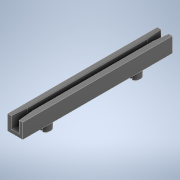
# Autodesk Inventor part: RDC-250
Saved by Autodesk Inventor 2021 (Build 250183000, 183)
## iProperties
Created: 2021-01-15
Part Number: RDC-250
Material: Nylon 6/6
Document SubType Name: Modeling
Designer: dimercur
Density: 1.13 g/cm^3
Appearance: Lisse - Noir
Author: dimercur
Autodesk Inventor part; units mm, degrees
ref_plane "YZ Plane" through (0, 0, 0) normal (1, 0, 0) x (0, 1, 0)
ref_plane "XZ Plane" through (0, 0, 0) normal (0, 1, 0) x (-1, 0, 0)
ref_plane "XY Plane" through (0, 0, 0) normal (0, 0, 1) x (1, 0, 0)
sketch "Esquisse1" plane through (0, 0, 0) normal (0, 1, 0) x (-1, 0, 0)
  line L0 (3.2, 31.75) -> (-3.2, 31.75)
  line L1 (-3.2, 31.75) -> (-3.2, -31.75)
  line L2 (-3.2, -31.75) -> (3.2, -31.75)
  line L3 (3.2, -31.75) -> (3.2, 31.75)
  point P0 (0, 0)
  dimension "d0" = 63.5
  dimension "d1" = 6.4
  dimension "d2" = 3.2
  dimension "d3" = 31.75
  constraints: 8 end point, 2 parallel, 1 horizontal, 1 perpendicular
  measures "d0" distance of L2.end L0.start
  measures "d1" distance of L0.start L0.end
  measures "d2" horizontal distance of point (0, 0) L0.start
  measures "d3" vertical distance of L0.start point (0, 0)
extrude "Extrusion1" add sketch "Esquisse1" along normal blind 6.4
sketch "Esquisse2" plane through (0, 6.4, 0) normal (0, 1, 0) x (1, 0, 0)
  line L0 (-3.2, -31.75) -> (3.2, -31.75) projected
  line L1 (-1.65, -31.75) -> (-1, -25.35)
  line L2 (-1, -25.35) -> (-1, 25.35)
  line L3 (-1, 25.35) -> (-1.65, 31.75)
  line L4 (3.2, 31.75) -> (-3.2, 31.75) projected
  line L5 (-1.65, 31.75) -> (1.65, 31.75)
  line L6 (1.65, 31.75) -> (1, 25.35)
  line L7 (1, 25.35) -> (1, -25.35)
  line L8 (1, -25.35) -> (1.65, -31.75)
  line L9 (1.65, -31.75) -> (-1.65, -31.75)
  point P0 (0, 0)
  dimension "d6" = 3.3
  dimension "d7" = 3.3
  dimension "d8" = 1.65
  dimension "d9" = 1.65
  dimension "d10" = 2
  dimension "d11" = 1
  dimension "d12" = 6.4
  dimension "d13" = 6.4
  dimension "d14" = 6.4
  dimension "d15" = 6.4
  constraints: 16 end point, 2 perpendicular, 2 point on line, 1 horizontal, 1 parallel
  measures "d6" distance of L8.end L1.start
  measures "d7" distance of L5.end L3.end
  measures "d8" horizontal distance of point (0, 0) L3.end
  measures "d9" horizontal distance of point (0, 0) L1.start
  measures "d10" distance between parallel lines of L7 L2
  measures "d11" horizontal distance of point (0, 0) L1.end
  measures "d12" vertical distance of L1.start L1.end
  measures "d13" vertical distance of L8.end L7.end
  measures "d14" vertical distance of L3.end L2.end
  measures "d15" vertical distance of L5.end L6.end
extrude "Extrusion2" cut sketch "Esquisse2" against normal blind 5.1
sketch "Esquisse3" plane through (0, 0, 0) normal (0, -1, 0) x (1, 0, 0)
  circle A0 centre (0, 19.05) radius 2.375
  circle A1 centre (0, -19.05) radius 2.375
  line L0 (-3.2, -31.75) -> (-3.2, 31.75) projected
  line L1 (3.2, 31.75) -> (3.2, -31.75) projected
  point P0 (0, 0)
  dimension "d18" = 4.75
  dimension "d19" = 19.05
  dimension "d20" = 38.1
  dimension "d21" = 4.75
  dimension "d22" = 6.4
  dimension "d23" = 3.2
  dimension "d24" = 3.2
  constraints: 2 centre point
  measures "d18" diameter of A0
  measures "d19" distance of point (0, 0) A0.centre
  measures "d20" distance of A1.centre A0.centre
  measures "d21" diameter of A1
  measures "d22" distance between parallel lines of L0 L1
  measures "d23" distance from line of L1 A0.centre
  measures "d24" distance from line of L1 A1.centre
extrude "Extrusion3" add sketch "Esquisse3" along normal blind 4.8
sketch "Esquisse4" plane through (0, -4.8, 19.05) normal (0, -1, 0) x (1, 0, 0)
  line L0 (-1, 6.3) -> (-1, -44.4) projected
  line L1 (1, 3.95) -> (-1, 3.95)
  line L2 (-1, 3.95) -> (-1, -4.05)
  line L3 (-1, -4.05) -> (1, -4.05)
  line L4 (1, -4.05) -> (1, 3.95)
  line L5 (1, -34.05) -> (-1, -34.05)
  line L6 (-1, -34.05) -> (-1, -42.05)
  line L7 (-1, -42.05) -> (1, -42.05)
  line L8 (1, -42.05) -> (1, -34.05)
  point P0 (0, -19.05)
  point P1 (-1, 3.95)
  dimension "d27" = 2
  dimension "d28" = 15
  dimension "d29" = 15
  dimension "d30" = 8
  dimension "d31" = 8
  constraints: 16 end point, 4 parallel, 3 point on line, 2 horizontal, 2 perpendicular
  measures "d27" distance of L2.end L3.end
  measures "d28" distance from line of point (0, -19.05) L3
  measures "d29" distance from line of point (0, -19.05) L5
  measures "d30" distance of L3.end L1.start
  measures "d31" distance of L7.end L5.start
extrude "Extrusion4" cut sketch "Esquisse4" against normal blind 4.8
chamfer "Chanfrein1" distance 1.3 angle 45 2 edges at (2.375, -4.8, 19.05) (-2.375, -4.8, 19.05)
chamfer "Chanfrein2" distance 1.3 angle 45 2 edges at (-2.375, -4.8, -19.05) (2.375, -4.8, -19.05)
equation "\"d2\" = 0.5 * d1"
equation "\"d3\" = 0.5 * d0"
equation "\"d7\" = d6"
equation "\"d8\" = 0.5 * d7"
equation "\"d9\" = 0.5 * d6"
equation "\"d11\" = 0.5 * d10"
equation "\"d13\" = d12"
equation "\"d14\" = d12"
equation "\"d15\" = d12"
equation "\"d19\" = 0.5 * d20"
equation "\"d21\" = d18"
equation "\"d23\" = 0.5 * d22"
equation "\"d24\" = d23"
